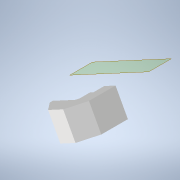
# Autodesk Inventor part: Matchboxscope_Lightperiscope_long_V0
Saved by Autodesk Inventor 2022 (Build 260153000, 153)
## iProperties
Created: 2022-03-26
Part Number: Matchboxscope_Lightperiscope_long_V0
Material: Generic
Document SubType Name: Modeling
Designer: Prakash Lab
Density: 1 g/cm^3
Appearance: Default
Author: Prakash Lab
Autodesk Inventor part; units mm, degrees
ref_plane "YZ Plane" through (0, 0, 0) normal (1, 0, 0) x (0, 1, 0)
ref_plane "XZ Plane" through (0, 0, 0) normal (0, 1, 0) x (-1, 0, 0)
ref_plane "XY Plane" through (0, 0, 0) normal (0, 0, 1) x (1, 0, 0)
ref_plane "Work Plane1" through (118.9518, 9.9874, -13.1749) normal (0.4728584, -0.8811384, 0) x (0, 0, -1)
sketch "Sketch1" plane through (118.9518, 9.9874, -13.1749) normal (0.4728584, -0.8811384, 0) x (0, 0, -1)
  line L0 (-16.5984, 5.5392) -> (-16.5984, 6.0404)
  line L1 (-1.2281, -14.4596) -> (-31.7652, -14.4596) construction
  line L2 (-16.5984, 11.5008) -> (-16.5984, -0.9971) projected
  line L3 (-15.5984, -2) -> (-12.5984, -2)
  line L4 (-16.5984, 2) -> (-12.5984, 2)
  line L5 (-16.5984, -3.9596) -> (-29.0984, -3.9596)
  line L6 (-29.0984, -3.9596) -> (-30.5984, -5.4596)
  line L7 (-30.5984, -5.4596) -> (-30.5984, -8.4596)
  line L8 (-30.5984, -8.4596) -> (-30.5984, -20.4596)
  line L9 (-30.5984, -20.4596) -> (-34.5984, -20.4596)
  line L10 (-34.5984, -20.4596) -> (-42.5984, -12.4596)
  line L11 (-42.5984, -12.4596) -> (-42.5984, -2.0772)
  line L12 (-42.5984, -2.0772) -> (-34.5984, 5.9228)
  line L13 (-34.5984, 5.9228) -> (-16.5984, 5.9228)
  line L14 (-16.5984, 0.8574) -> (-16.5984, 5.9228)
  line L15 (-16.5984, 2.0404) -> (-48.439, 2.0404) construction
  line L16 (-16.5984, -0.9971) -> (-16.5984, -3.9596)
  line L17 (-16.5984, -0.0772) -> (-40.5984, -0.0772) construction
  line L18 (-40.5984, -0.0772) -> (-40.5984, -14.4596) construction
  line L19 (-16.5984, -0.0772) -> (-40.5984, -0.0772)
  point P0 (-13.1749, -109.5356)
  point P1 (-16.5984, 0.8574)
  dimension "d25" = 135
  dimension "d26" = 4
  dimension "d27" = 6
  dimension "d28" = 3.8824
  dimension "d29" = 6
  dimension "d31" = 12
  dimension "d40" = 1.5
  dimension "d42" = 26
  dimension "d45" = 0
  dimension "d50" = 8
  dimension "d51" = 10
  dimension "d52" = 16.5
  constraints: 38 end point, 7 point on line, 6 horizontal, 5 perpendicular, 4 collinear, 2 parallel, 4 other
  measures "d25" angle of L9 L10
  measures "d26" distance between parallel lines of L4 L3
  measures "d27" distance between parallel lines of L5 L15
  measures "d28" distance between parallel lines of L13 L15
  measures "d29" distance between parallel lines of L9 L1
  measures "d31" distance between parallel lines of L7 L11
  measures "d40" horizontal distance of L5.end L6.end
  measures "d42" distance between parallel lines of L16 L11
  measures "d45" horizontal distance of L12.end L9.end
  measures "d50" distance from line of L9.end L11
  measures "d51" distance of L0.end L5.start
  measures "d52" distance between parallel lines of L5 L9
extrude "Extrusion1" add sketch "Sketch1" along normal blind 1.5
sketch "Sketch2" plane through (119.6611, 8.6657, -13.1749) normal (0.4728584, -0.8811384, 0) x (0.8811384, 0.4728584, 0)
  line L0 (-2.0772, 42.5984) -> (-12.4596, 42.5984) projected
  line L1 (-12.4596, 42.5984) -> (-20.4596, 34.5984) projected
  line L2 (-20.4596, 34.5984) -> (-20.4596, 30.5984) projected
  line L3 (-20.4596, 30.5984) -> (-5.4596, 30.5984) projected
  line L4 (-5.4596, 30.5984) -> (-3.9596, 29.0984) projected
  line L5 (-3.9596, 29.0984) -> (-3.9596, 16.5984) projected
  line L6 (5.9228, 16.5984) -> (5.9228, 34.5984) projected
  line L7 (5.9228, 34.5984) -> (-2.0772, 42.5984) projected
  line L8 (-3.9596, 16.5984) -> (5.9228, 16.5984) projected
  line L9 (-11.8383, 41.0984) -> (-2.6985, 41.0984)
  line L10 (-2.6985, 41.0984) -> (4.4228, 33.9771)
  line L11 (4.4228, 33.9771) -> (4.4228, 18.0984)
  line L12 (4.4228, 18.0984) -> (-0.9902, 18.0984)
  line L13 (-0.9902, 18.0984) -> (-2.3894, 18.1112)
  line L14 (-2.3894, 18.1112) -> (-2.3894, 29.7488)
  line L15 (-2.3894, 29.7488) -> (-4.8092, 32.1686)
  line L16 (-4.8092, 32.1686) -> (-8.9884, 32.1686)
  line L17 (-8.9884, 32.1686) -> (-9.9596, 32.1686)
  line L18 (-9.9596, 32.1686) -> (-18.9596, 32.1686)
  line L19 (-18.9596, 32.1686) -> (-18.9596, 33.9771)
  line L20 (-18.9596, 33.9771) -> (-11.8383, 41.0984)
  point P0 (-109.5356, 13.1749)
  dimension "d41" = 1.5
  constraints: 24 end point, 1 horizontal, 6 other
  measures "d41" distance between parallel lines of L0 L9
extrude "Extrusion2" add sketch "Sketch2" along normal blind 14
sketch "Sketch3" plane through (103.6773, 1.7904, 17.4235) normal (0, 0, -1) x (-0.8811384, -0.4728584, 0)
  circle A0 centre (-2.8052, -7.75) radius 4.5
  line L0 (3.1948, 0) -> (-8.8052, 0) projected
  line L1 (-8.8052, 0) -> (-8.8052, -15.5) projected
  line L2 (3.1948, -15.5) -> (-8.8052, -15.5) projected
  line L3 (3.1948, 0) -> (3.1948, -15.5) projected
  point P0 (92.2006, 47.4471)
  constraints: 1 centre point
extrude "Extrusion3" cut sketch "Sketch3" against normal blind 1.5 contours A0
sketch "Sketch8" plane through (119.7213, 8.698, 3.4235) normal (0, 0, 1) x (0.8811384, 0.4728584, 0)
  circle A0 centre (-19.1075, 3.6497) radius 1.4001 projected
  circle A1 centre (-14.1578, 7.8923) radius 2 projected
  circle A2 centre (-14.1578, 7.8923) radius 3.3708
  point P0 (-109.604, 48.9471)
  constraints: 1 centre point
extrude "Extrusion8" cut sketch "Sketch8" along normal mid plane 14 contours A1 | A2
sketch "Sketch9" plane through (118.7885, 8.1974, 4.9235) normal (0, 0, 1) x (0.8811384, 0.4728584, 0)
  circle A0 centre (0.9902, -6.25) radius 1.352 projected
  circle A1 centre (0.9902, -6.25) radius 2.6601
  point P0 (-108.5454, 48.9471)
  constraints: 1 centre point, 1 coincident
extrude "Extrusion9" cut sketch "Sketch9" along normal mid plane 14 contours A0 | A1
sketch "Skizze11" plane through (118.9518, 9.9874, -13.1749) normal (-0.4728584, 0.8811384, 0) x (0.8811384, 0.4728584, 0)
  line L0 (-2.0772, -42.5984) -> (-12.4596, -42.5984) projected
  line L1 (5.9228, -34.5984) -> (-2.0772, -42.5984) projected
  line L2 (5.9228, -16.5984) -> (5.9228, -34.5984) projected
  line L3 (-3.9596, -16.5984) -> (5.9228, -16.5984) projected
  line L4 (-3.9596, -29.0984) -> (-3.9596, -16.5984) projected
  line L5 (-5.4596, -30.5984) -> (-3.9596, -29.0984) projected
  line L6 (-20.4596, -30.5984) -> (-5.4596, -30.5984) projected
  line L7 (-20.4596, -34.5984) -> (-20.4596, -30.5984) projected
  line L8 (-12.4596, -42.5984) -> (-20.4596, -34.5984) projected
  line L9 (-3.9596, -16.5984) -> (5.9228, -16.5984) projected
  line L10 (-3.9596, -29.0984) -> (-3.9596, -16.5984) projected
  line L11 (-1.6499, -16.5984) -> (-3.9596, -16.5984)
  line L12 (-3.9596, -16.5984) -> (-3.9596, -26.5984)
  line L13 (-3.9596, -26.5984) -> (-1.6499, -26.5984)
  line L14 (-1.6499, -26.5984) -> (-1.6499, -16.5984)
  point P0 (-109.5356, -13.1749)
  point P1 (-3.9596, -26.5984)
  dimension "d57" = 10
  constraints: 8 end point, 2 parallel, 2 point on line, 1 horizontal, 1 perpendicular
  measures "d57" distance between parallel lines of L13 L3
extrude "Extrusion11" cut sketch "Skizze11" against normal through all contours L14 L13 L4 L3
sketch "Skizze12" plane through (119.6611, 8.6657, -13.1749) normal (0.4728584, -0.8811384, 0) x (0.8811384, 0.4728584, 0)
  line L0 (-2.3894, 26.5984) -> (-1.6499, 26.5984) projected
  line L1 (-1.6499, 26.5984) -> (-1.6499, 18.1045) projected
  line L2 (-1.6499, 18.1045) -> (-0.9902, 18.0984) projected
  line L3 (-0.9902, 18.0984) -> (4.4228, 18.0984) projected
  line L4 (4.4228, 18.0984) -> (4.4228, 33.9771) projected
  line L5 (4.4228, 33.9771) -> (-2.6985, 41.0984) projected
  line L6 (-2.6985, 41.0984) -> (-11.8383, 41.0984) projected
  line L7 (-11.8383, 41.0984) -> (-18.9596, 33.9771) projected
  line L8 (-18.9596, 33.9771) -> (-18.9596, 32.1686) projected
  line L9 (-18.9596, 32.1686) -> (-4.8092, 32.1686) projected
  line L10 (-4.8092, 32.1686) -> (-2.3894, 29.7488) projected
  line L11 (-2.3894, 29.7488) -> (-2.3894, 26.5984) projected
  line L12 (-3.9596, 26.5984) -> (-2.3894, 26.5984) projected
  line L13 (-2.3894, 26.5984) -> (-1.6499, 26.5984)
  line L14 (-1.6499, 26.5984) -> (-1.6499, 27.0984)
  line L15 (-1.6499, 27.0984) -> (-2.3894, 27.0984)
  line L16 (-2.3894, 27.0984) -> (-2.3894, 26.5984)
  line L17 (-0.9902, 18.0984) -> (4.4228, 18.0984) projected
  line L18 (-1.6499, 27.0984) -> (-1.1499, 27.0984)
  line L19 (-1.1499, 27.0984) -> (-1.1499, 18.0984)
  line L20 (-1.1499, 18.0984) -> (-1.6499, 18.0984)
  line L21 (-1.6499, 18.0984) -> (-1.6499, 27.0984)
  line L22 (-1.6499, 18.1045) -> (-0.9902, 18.0984) projected
  line L23 (-1.6499, 16.5984) -> (5.9228, 16.5984) projected
  line L24 (-1.6499, 18.1045) -> (-1.1499, 18.1045)
  line L25 (-1.1499, 18.1045) -> (-1.1499, 16.5984)
  line L26 (-1.1499, 16.5984) -> (-1.6499, 16.5984)
  line L27 (-1.6499, 16.5984) -> (-1.6499, 18.1045)
  point P0 (-109.5356, 13.1749)
  point P1 (-2.3894, 27.0984)
  point P2 (-1.1499, 18.0999)
  point P3 (-1.6499, 18.0984)
  point P4 (-1.1499, 18.0984)
  dimension "d53" = 0.5
  dimension "d54" = 0.5
  constraints: 24 end point, 6 parallel, 3 horizontal, 3 perpendicular, 2 point on line
  measures "d53" distance of L14.end L13.end
  measures "d54" distance between parallel lines of L19 L21
extrude "Extrusion12" add sketch "Skizze12" along normal up to surface (14 mm away) contours L11 L15 L14 L0 | L14 L18 L19 L24 L1 | L24 L19 L2 | L25 L23 L27 L20
body "Solid1"
